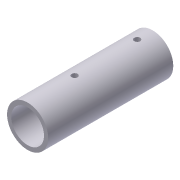
# Autodesk Inventor part: FE-00018-02
Saved by Autodesk Inventor 2012 (Build 160160000, 160)
## iProperties
Company: FIRST
Created: 2008-05-30
Part Number: FE-00018-02
Document SubType Name: Modeling
Designer: dfoster
Density: 1 g/cm^3
Description: Insert Tube
Mass: 32.1332 g
Surface Area: 198.679 cm^2
Volume: 32.1332 cm^3
Material: Default
Title: Insert Tube
Author: dfoster
Autodesk Inventor part; units mm, degrees
ref_plane "XZ Plane" through (0, 0, 0) normal (0, 1, 0) x (-1, 0, 0)
ref_plane "XY Plane" through (0, 0, 0) normal (0, 0, 1) x (1, 0, 0)
sketch "Sketch1" plane through (0, 0, 0) normal (0, 0, 1) x (1, 0, 0)
  circle A0 centre (0, 0) radius 16.7005
  circle A1 centre (0, 0) radius 13.3223
  dimension "d0" = 26.6446
  dimension "d1" = 33.401
  constraints: 2 centre point, 1 coincident
  measures "d0" diameter of A1
  measures "d1" diameter of A0
extrude "Extrusion1" add sketch "Sketch1" along normal blind 101.6
ref_plane "Work Plane1" through (0, 0, 0) normal (0, 1, 0) x (0, 0, 1)
sketch "Sketch2" plane through (0, 0, 0) normal (0, 1, 0) x (0, 0, 1)
  line L0 (0, -16.7005) -> (101.6, -16.7005) projected
  line L1 (101.6, 13.3223) -> (101.6, -13.3223) projected
  line L2 (101.6, 16.7005) -> (101.6, -16.7005) projected
  line L3 (-20.32, 0) -> (121.92, 0) projected
  circle A0 centre (63.5, 0) radius 2.4257
  dimension "d5" = 38.1
  dimension "d6" = 4.8514
  constraints: 1 centre point, 1 point on line
  measures "d5" distance from line of L2 A0.centre
  measures "d6" diameter of A0
extrude "Extrusion2" cut sketch "Sketch2" against normal mid plane 1638.3
pattern_linear "Rectangular Pattern1" count 2 spacing 50.8 along (0, 0, -1) of "Extrusion2"
body "Solid1"
